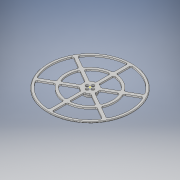
# Autodesk Inventor part: fly
Saved by Autodesk Inventor 2018 (Build 220112000, 112)
## iProperties
Created: 2019-11-23
Part Number: fly
Material: Generic
Document SubType Name: Modeling
Designer: Bunny320
Density: 1 g/cm^3
Appearance: Default
Author: Bunny320
## iProperties of the stored document fly_3DPrint.ipt
Created: 2019-11-23
Part Number: fly_3DPrint
Material: Generic
Document SubType Name: Modeling
Designer: Bunny320
Density: 1 g/cm^3
Appearance: Default
Author: Bunny320
Autodesk Inventor part; units mm, degrees
ref_plane "YZ Plane" through (0, 0, 0) normal (1, 0, 0) x (0, 1, 0)
ref_plane "XZ Plane" through (0, 0, 0) normal (0, 1, 0) x (-1, 0, 0)
ref_plane "XY Plane" through (0, 0, 0) normal (0, 0, 1) x (1, 0, 0)
sketch "Sketch1" plane through (0, 0, 0) normal (0, 0, 1) x (1, 0, 0)
  circle A0 centre (0, 0) radius 85
  dimension "d0" = 170
  constraints: 1 centre point, 1 coincident
  measures "d0" diameter of A0
extrude "Extrusion1" add sketch "Sketch1" along normal blind 9
sketch "Sketch2" plane through (0, 0, 9) normal (0, 0, 1) x (1, 0, 0)
  point P0 (0, 0)
  point P1 (6, 0)
  dimension "d3" = 6
  measures "d3" distance of point (0, 0) point (6, 0)
hole "Hole1" at (6, 0, 9) direction (0, 0, -1) diameter 3.4 end through all counterbore diameter 6 counterbore depth 3 clearance for "Hex Head Cap Screw DIN EN 24017" size "M3" standard "DIN"
pattern_circular "Circular Pattern1" count 4 over 360 about axis through (0, 0, -10) along (0, 0, 1) of "Hole1"
sketch "Sketch3" plane through (0, 0, 0) normal (0, 0, 1) x (1, 0, 0)
  circle A0 centre (0, 0) radius 12.5
  circle A1 centre (0, 0) radius 85
  dimension "d14" = 25
  constraints: 2 centre point, 2 coincident
  measures "d14" diameter of A0
extrude "Extrusion2" cut sketch "Sketch3" along normal blind 6
sketch "Sketch4" plane through (0, 0, 9) normal (0, 0, 1) x (1, 0, 0)
  circle A0 centre (0, 0) radius 15
  circle A1 centre (0, 0) radius 80
  circle A2 centre (0, 0) radius 45
  circle A3 centre (0, 0) radius 50
  dimension "d18" = 30
  dimension "d19" = 160
  dimension "d22" = 90
  dimension "d23" = 100
  constraints: 4 centre point, 4 coincident
  measures "d18" diameter of A0
  measures "d19" diameter of A1
  measures "d22" diameter of A2
  measures "d23" diameter of A3
sketch "Sketch5" plane through (0, 0, 9) normal (0, 0, 1) x (1, 0, 0)
  point P0 (0, 0)
extrude "Extrusion4" cut sketch "Sketch4" against normal through all
sketch "Sketch6" plane through (0, 0, 9) normal (0, 0, 1) x (1, 0, 0)
  line L0 (3, 81.5322) -> (-3, 81.5322)
  line L1 (-3, 81.5322) -> (-3, 11.5322)
  line L2 (-3, 11.5322) -> (3, 11.5322)
  line L3 (3, 11.5322) -> (3, 81.5322)
  line L4 (3, 81.5322) -> (-3, 11.5322) construction
  line L5 (-3, 81.5322) -> (3, 11.5322) construction
  point P0 (0, 0)
  point P1 (0, 46.5322)
  dimension "d26" = 6
  dimension "d30" = 70
  constraints: 12 end point, 2 midpoint, 2 parallel, 1 horizontal, 1 perpendicular
  measures "d26" distance of L1.end L2.end
  measures "d30" distance of L0.end L1.end
extrude "Extrusion5" add sketch "Sketch6" against normal blind 3
fillet "Fillet2" radius 3 8 edges at (-3, 14.6969, 7.5) (-3, 44.8999, 7.5) (-3, 49.9099, 7.5) (-3, 79.9437, 7.5) (3, 79.9437, 7.5) (3, 49.9099, 7.5) (3, 44.8999, 7.5) (3, 14.6969, 7.5)
pattern_circular "Circular Pattern2" count 6 over 360 about axis through (0, 0, -10) along (0, 0, 1) of "Extrusion5", "Fillet2"
fillet "Fillet1" radius 1 2 edges at (-85, 0, 9) (-85, 0, 6)
body "Solid1"
